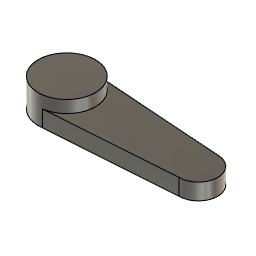
Filter v36 (Autodesk Fusion 360 archive; units mm, degrees)
design "ServoArm"
Autodesk Fusion 360 part; units mm, degrees
cylinder "CylinderPrimitive1" add diameter 7 height 3.5 placed x (1, 0, 0) y (0, 1, 0) z (0, 0, 1) at (0, 0, 0) makes body 1
cylinder "CylinderPrimitive2" add diameter 4.75 height 2 placed x (1, 0, 0) y (0, 1, 0) z (0, 0, 1) at (17.5, 0, 0) separate body makes body 2
move_face "MoveFace1" to x (1, 0, 0) y (0, 1, 0) z (0, 0, 1) at (3.5, 0, 0) 1 faces at (3.4826, -0.3485, 1.1667) on bodies 1
move_face "MoveFace2" to x (1, 0, 0) y (0, 1, 0) z (0, 0, 1) at (2.125, 0, 0) 1 faces at (19.8632, -0.2365, 1.3333) on bodies 2
sketch "Sketch3" plane through (0, 0, 0) normal (0, 0, 1) x (1, 0, 0)
  line L0 (19.625, -2.375) -> (3.5, -3.5)
  line L1 (3.5, -3.5) -> (3.5, 0)
  line L2 (3.5, 0) -> (19.6, 0)
  line L3 (19.6, 0) -> (19.625, -2.375)
  constraint vertical L1
  constraint perpendicular L1 L2
extrude "Extrude1" add sketch "Sketch3" along normal blind 2 separate body makes body 3
mirror "Mirror1" about plane through (0, 0, 0) normal (0, 1, 0) of bodies 3 merged
combine "Combine1" operation add target body 1 tool bodies 2 3
